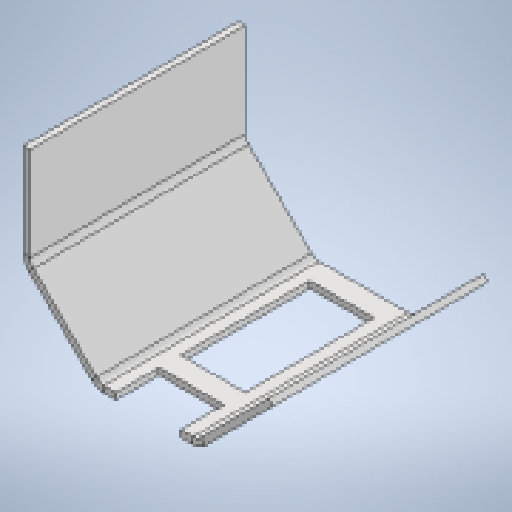
# Autodesk Inventor part: DS-B-101 Axis
Saved by Autodesk Inventor 2025.1 (Build 291241020, 241B)
## iProperties
Created: 2025-01-13
Part Number: DS-B-101 Axis
Material: Stainless Steel
Document SubType Name: Sheet Metal
Designer: Dobrov
Mass: 256.049 g
Surface Area: 335.823 cm^2
Volume: 32.0061 cm^3
Density: 8 g/cm^3
Sheet Metal Rule: AISI304 3mm Die 32
Sheet Metal Width: 100.000 mm
Sheet Metal Length: 183.009 mm
Sheet Metal Area: 18300.890 mm^2
Appearance: Default
Flat Pattern Width: 10 cm
Flat Pattern Length: 18.3009 cm
Flat Pattern Area: 183.009 cm^2
Author: user
Autodesk Inventor part; units mm, degrees
ref_plane "YZ Plane" through (0, 0, 0) normal (1, 0, 0) x (0, 1, 0)
ref_plane "XZ Plane" through (0, 0, 0) normal (0, 1, 0) x (-1, 0, 0)
ref_plane "XY Plane" through (0, 0, 0) normal (0, 0, 1) x (1, 0, 0)
sketch "Sketch1" plane through (0, 0, 0) normal (0, 0, 1) x (1, 0, 0)
  line L0 (-23.5, -50) -> (23.5, -50)
  line L1 (23.5, -50) -> (23.5, 50)
  line L2 (23.5, 50) -> (-23.5, 50)
  line L3 (-23.5, 50) -> (-23.5, -50)
  line L4 (-23.5, -50) -> (23.5, 50) construction
  line L5 (23.5, -50) -> (-23.5, 50) construction
  point P0 (0, 0)
  dimension "d154" = 47
  dimension "d155" = 100
  measures "d154" distance of L1.end L2.end
  measures "d155" distance of L0.end L1.end
extrude "Plate3" add sketch "Sketch1" along normal blind 3
sketch "Sketch7" plane through (21.3787, 50, 2.1213) normal (0.7071068, 0, -0.7071068) x (0, 1, 0)
  line L0 (-100, 0) -> (0, 0)
  line L1 (0, 0) -> (0, 47)
  line L2 (0, 47) -> (-100, 47)
  line L3 (-100, 47) -> (-100, 0)
  constraints: 6 end point, 1 horizontal, 1 perpendicular, 1 vertical
edge flange "Flange3" height 47 angle 45 thickness 3 bend radius 5 thickness toward (0.7071068, 0, -0.7071068) relief round relief width 3 relief depth 1.5 corner gap 5 corner form 0 edges at (23.5, 0, 3) (-23.5, 0, 3) wall of the first edge with corners at (21.3787, -50, 2.1213) (21.3787, 50, 2.1213) (54.6127, 50, 35.3553) (54.6127, -50, 35.3553)
bend "Bend3"
corner "Corner3"
sketch "Sketch8" plane through (0, 0, 3) normal (0, 0, 1) x (1, 0, 0)
  line L0 (15, 40) -> (-15, 40)
  line L1 (-15, 40) -> (-15, -20)
  line L2 (-15, -20) -> (15, -20)
  line L3 (15, -20) -> (15, 40)
  line L4 (15, 40) -> (-15, -20) construction
  line L5 (-15, 40) -> (15, -20) construction
  line L6 (-23.5, 50) -> (20.1863, 50) projected
  line L7 (-20.1863, -50) -> (20.1863, -50) projected
  line L8 (15, -50) -> (-15, -50)
  line L9 (-15, -50) -> (-15, -30)
  line L10 (-15, -30) -> (15, -30)
  line L11 (15, -30) -> (15, -50)
  point P0 (0, 0)
  point P1 (0, 10)
  point P2 (-15, -50)
  dimension "d166" = 30
  dimension "d168" = 10
  dimension "d182" = 10
  dimension "d183" = 20
  constraints: 20 end point, 4 parallel, 2 collinear, 2 horizontal, 2 midpoint, 2 perpendicular, 1 point on line, 1 vertical alignment
  measures "d166" distance of L2.end L1.end
  measures "d168" distance between parallel lines of L0 L6
  measures "d182" distance between parallel lines of L10 L2
  measures "d183" distance of L8.end L9.end
extrude "Cut1" cut sketch "Sketch8" against normal blind 3
sketch "Sketch9" plane through (-53.734, -50, 33.234) normal (-1, 0, 0) x (0, -1, 0)
  line L0 (-100, 0) -> (0, 0)
  line L1 (0, 0) -> (0, 47)
  line L2 (0, 47) -> (-100, 47)
  line L3 (-100, 47) -> (-100, 0)
  constraints: 6 end point, 1 horizontal, 1 perpendicular, 1 vertical
edge flange "Flange4" height 47 angle 45 thickness 3 bend radius 5 thickness toward (-1, 0, 0) relief round relief width 3 relief depth 1.5 edges at (-54.6127, 0, 35.3553) wall of the first edge with corners at (-53.734, 50, 33.234) (-53.734, -50, 33.234) (-53.734, -50, 80.234) (-53.734, 50, 80.234)
bend "Bend4"
corner "Corner4"
body "Solid2"
